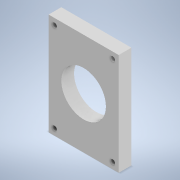
# Autodesk Inventor part: Encoder Mount Y
Saved by Autodesk Inventor 2020 (Build 240168000, 168)
## iProperties
Created: 2020-03-20
Part Number: Encoder Mount Y
Material: Generic
Document SubType Name: Modeling
Designer: DasNick
Density: 1 g/cm^3
Appearance: Default
Author: DasNick
Autodesk Inventor part; units mm, degrees
ref_plane "YZ Plane" through (0, 0, 0) normal (1, 0, 0) x (0, 1, 0)
ref_plane "XZ Plane" through (0, 0, 0) normal (0, 1, 0) x (-1, 0, 0)
sketch "Sketch1" plane through (0, 0, 0) normal (0, 0, 1) x (1, 0, 0)
  line L0 (34.925, 95.25) -> (-34.925, 95.25) projected
  line L1 (-34.925, 95.25) -> (-34.925, 82.55) projected
  line L2 (-34.925, 82.55) -> (34.925, 82.55) projected
  line L3 (34.925, 82.55) -> (34.925, 95.25) projected
  circle A0 centre (-29.0032, 88.9) radius 2.3812 projected
  circle A1 centre (29.0032, 88.9) radius 2.3812 projected
  line L4 (34.925, 6.35) -> (-34.925, 6.35) projected
  line L5 (-34.925, 6.35) -> (-34.925, -6.35) projected
  line L6 (-34.925, -6.35) -> (34.925, -6.35) projected
  line L7 (34.925, -6.35) -> (34.925, 6.35) projected
  circle A2 centre (-29.0032, 0) radius 2.3812 projected
  circle A3 centre (29.0032, 0) radius 2.3812 projected
  line L8 (34.925, 82.55) -> (34.925, 6.35)
  line L9 (-34.925, 6.35) -> (-34.925, 82.55)
  circle A4 centre (0, 44.45) radius 22.225
  point P0 (0, 0)
  dimension "d0" = 44.45
  constraints: 4 end point, 1 centre point, 1 parallel, 1 vertical
  measures "d0" diameter of A4
extrude "Extrusion1" add sketch "Sketch1" along normal blind 12.7
ref_plane "Work Plane1" through (-19.4127, 25.0373, 33.395) normal (0, 0, -1) x (0, 1, 0)
body "Solid1"
